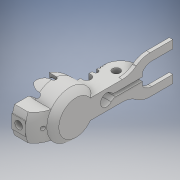
# Autodesk Inventor part: NeuroprobeholdermajigerV11MiniscopeAngle43DScope
Saved by Autodesk Inventor 2017 (Build 210142000, 142)
## iProperties
Created: 2017-09-22
Part Number: NeuroprobeholdermajigerV11MiniscopeAngle43DScope
Material: Generic
Document SubType Name: Modeling
Designer: andrew
Density: 1 g/cm^3
Appearance: Default
Author: andrew
Autodesk Inventor part; units mm, degrees
ref_plane "YZ Plane" through (0, 0, 0) normal (1, 0, 0) x (0, 1, 0)
sketch "Sketch2" plane through (0, 0, 0) normal (0, 0, 1) x (1, 0, 0)
  arc A0 (10.5, 0) -> (-2.9904, 10.0652) centre (0, 0) ccw
  arc A1 (0, 12) -> (-6, 10.3923) centre (0, 0) ccw
  line L0 (-5.25, 9.0933) -> (-6, 10.3923)
  line L1 (0, 0) -> (17.0475, 0) construction
  line L2 (0, 0) -> (-8.3214, 0)
  line L3 (11.5, 0) -> (0, 0)
  line L4 (0, 12) -> (8.279, 12)
  line L5 (11.5, 8.9606) -> (11.5, 0)
  line L6 (8.279, 12) -> (7.279, 12)
  line L7 (7.279, 12) -> (8.279, 12)
  arc A2 (11.5, 8.9606) -> (8.279, 12) centre (0, 0) ccw
  arc A3 (-5.25, 9.0933) -> (-4.1869, 9.0866) centre (-4.7167, 9.3682) ccw
  arc A4 (-2.9904, 10.0652) -> (-4.1869, 9.0866) centre (-2.4208, 8.148) ccw
  point P0 (-8.5237, 14.7636)
  point P1 (-8.5237, -14.7636)
  dimension "d5" = 24
  dimension "d6" = 120
  dimension "d75" = 2
  constraints: 16 end point, 10 point on circle, 5 centre point, 3 coincident, 3 horizontal, 3 point on line, 2 tangent, 1 collinear, 1 perpendicular, 1 symmetric about line
  measures "d5" diameter of A1
  measures "d6" angle of L1 L0
  measures "d75" radius of A4
revolve "Revolution2" add sketch "Sketch2" angle 360 about axis through (0, 0, 0) along (-1, 0, 0)
sketch "Sketch1" plane through (0, 0, 0) normal (0, 1, 0) x (-1, 0, 0)
  arc A0 (-10, 0) -> (9.4843, -3.17) centre (0, 0) ccw
  line L0 (0, 0) -> (0, -3.17)
  line L1 (9.4843, -3.17) -> (37.7274, -3.17)
  line L2 (0, 0) -> (4.0481, 0)
  line L3 (4.0481, 0) -> (4.0481, 0)
  line L4 (37.7274, 0) -> (37.7274, -3.17)
  line L5 (37.7274, 0) -> (-10, 0)
  point P0 (37.7274, 3.17)
  dimension "d0" = 20
  dimension "d1" = 3.17
  dimension "d2" = 90
  constraints: 12 end point, 2 perpendicular, 2 point on circle, 1 centre point, 1 coincident, 1 horizontal, 1 point on line, 1 symmetric about line, 1 vertical
  measures "d0" diameter of A0
  measures "d1" distance of L0.start L0.end
  measures "d2" angle of L1 L0
revolve "Revolution1" [suppressed]
sketch "Sketch4" plane through (0, 0, 0) normal (0, 1, 0) x (-1, 0, 0)
  line L0 (6.0157, -10.3923) -> (6.0157, 10.3923)
  line L1 (6.0157, -3.519) -> (6.0157, 3.519)
  line L2 (6, 0) -> (6, 0) construction
  line L3 (0.822, 9.7784) -> (0.822, -9.9241) construction
  arc A0 (0.0051, 1.2595) -> (6.0157, 3.519) centre (-0.0738, 10.5936) ccw
  arc A1 (-3.157, 1.9433) -> (-2.378, 1.548) centre (-1.8843, 3.4861) ccw
  arc A2 (0.0051, 1.2595) -> (0.0051, -1.2595) centre (0.0157, 0) ccw
  line L4 (-4.7599, 0) -> (0.0157, 0) construction
  arc A3 (-2.378, -1.548) -> (-3.157, -1.9433) centre (-1.8843, -3.4861) ccw
  arc A4 (6.0157, -3.519) -> (0.0051, -1.2595) centre (-0.0738, -10.5936) ccw
  line L5 (0.0157, 0) -> (-9.5355, 0) construction
  arc A5 (-3.157, 1.9433) -> (-3.157, -1.9433) centre (-4.7599, 0) ccw
  line L6 (11.1937, 0) -> (13.2584, 0)
  point P0 (0, 0)
  constraints: 12 end point, 12 point on circle, 6 centre point, 2 coincident, 1 collinear, 1 horizontal, 1 point on line, 1 vertical
extrude "Extrusion2" cut sketch "Sketch4" along normal blind 25
pattern_circular "Circular Pattern1" count 4 over 360 about axis through (-10, 0, 0) along (1, 0, 0) of "Extrusion2"
ref_plane "Work Plane1" through (0, -12, 0) normal (0, 1, 0) x (-1, 0, 0)
sketch "Sketch7" plane through (0, -12, 0) normal (0, 1, 0) x (-1, 0, 0)
  circle A0 centre (0, 0) radius 2.0066
  line L0 (-8.2285, 6.985) -> (3.5053, 6.985)
  line L1 (-8.279, -6.985) -> (3.5053, -6.985)
  line L2 (3.5053, -4.064) -> (-1.7598, -4.064)
  line L3 (-4.3994, -2.54) -> (-1.7598, -4.064)
  line L4 (-4.3994, 2.54) -> (-4.3994, -2.54)
  line L5 (-1.7598, 4.064) -> (-4.3994, 2.54)
  line L6 (-1.7598, 4.064) -> (3.5053, 4.064)
  circle A1 centre (0, 0) radius 2.0066
  line L7 (3.5053, 0.0727) -> (3.5053, 21.7197)
  line L8 (3.5053, 21.7197) -> (3.5053, -17.1959)
  line L9 (-8.279, -6.985) -> (-8.279, 6.985)
  line L10 (-8.2285, 6.985) -> (-8.279, 6.985)
  point P0 (0, 0)
  point P1 (0, 0)
  constraints: 22 end point, 5 point on line, 2 centre point
extrude "Extrusion4" add sketch "Sketch7" along normal blind 1.5
sketch "Sketch8" plane through (0, -10.5, 0) normal (0, 1, 0) x (1, 0, 0)
  line L0 (0, -5.8095) -> (8.279, -5.8095) projected
  arc A0 (-3.5053, -4.6328) -> (0, -5.8095) centre (0, 0) ccw projected
  line L1 (-3.5053, -4.6328) -> (-3.5053, -6.985) projected
  line L2 (-3.5053, -6.985) -> (8.279, -6.985) projected
  line L3 (8.279, 5.8095) -> (0, 5.8095) projected
  line L4 (8.279, 6.985) -> (-3.5053, 6.985) projected
  line L5 (-3.5053, 6.985) -> (-3.5053, 4.6328) projected
  arc A1 (0, 5.8095) -> (-3.5053, 4.6328) centre (0, 0) ccw projected
  line L6 (8.279, 5.8095) -> (8.279, 6.985) projected
  line L7 (8.279, -6.985) -> (8.279, -5.8095) projected
extrude "Extrusion5" add sketch "Sketch8" along normal blind 1.5
sketch "Sketch9" plane through (0, -12, 0) normal (0, -1, 0) x (1, 0, 0)
  circle A0 centre (0, 0) radius 2.0066
  line L0 (-3.5053, 6.985) -> (3.5053, 6.985)
  line L1 (-3.5053, -6.985) -> (3.5053, -6.985)
  line L2 (1.7598, -4.064) -> (-1.7598, -4.064)
  line L3 (-1.7598, 4.064) -> (1.7598, 4.064)
  circle A1 centre (0, 0) radius 2.0066
  circle A2 centre (0, 0) radius 2.0066
  line L4 (5.4916, 6.985) -> (-3.5053, 6.985)
  line L5 (5.4916, -6.985) -> (-3.5053, -6.985)
  line L6 (-3.5053, -4.064) -> (1.7598, -4.064)
  line L7 (4.3994, -2.54) -> (1.7598, -4.064)
  line L8 (4.3994, 2.54) -> (4.3994, -2.54)
  line L9 (1.7598, 4.064) -> (4.3994, 2.54)
  line L10 (1.7598, 4.064) -> (-3.5053, 4.064)
  circle A3 centre (0, 0) radius 2.0066
  line L11 (-3.5053, 0.0727) -> (-3.5053, 6.985)
  line L12 (-3.5053, 6.985) -> (-3.5053, -6.985)
  line L13 (8.279, 6.985) -> (5.6673, 6.985)
  line L14 (-3.5053, 6.985) -> (8.279, 6.985) projected
  line L15 (8.279, -6.985) -> (-3.5053, -6.985) projected
  line L16 (5.4916, -6.985) -> (8.279, -6.985)
  line L17 (8.279, 6.985) -> (8.279, -6.985)
  point P0 (0, 0)
  point P1 (0, 0)
  point P2 (-3.5053, -17.1959)
  constraints: 32 end point, 5 point on line, 4 centre point, 1 horizontal, 1 vertical
extrude "Extrusion6" add sketch "Sketch9" along normal blind 3.302 contours L0 L4 L14 L13 L17 L15 L5 L1 L12 L6 L2 L7 L8 L9 L3 L10 L11
sketch "Sketch10" plane through (0, -15.302, 0) normal (0, -1, 0) x (1, 0, 0)
  circle A0 centre (0, 0) radius 2.0066
  line L0 (-3.5053, 6.985) -> (3.5053, 6.985)
  line L1 (-3.5053, -6.985) -> (3.5053, -6.985)
  line L2 (1.7598, -4.064) -> (-1.7598, -4.064)
  line L3 (-1.7598, 4.064) -> (1.7598, 4.064)
  circle A1 centre (0, 0) radius 2.0066
  line L4 (-3.5053, 0.0727) -> (-3.5053, 6.985)
  line L5 (1.7598, 4.064) -> (-3.5053, 4.064)
  line L6 (1.7598, 4.064) -> (4.3994, 2.54)
  line L7 (5.4916, 6.985) -> (-3.5053, 6.985)
  line L8 (-3.5053, 6.985) -> (-3.5053, -6.985)
  circle A2 centre (0, 0) radius 2.0066
  line L9 (4.3994, 2.54) -> (4.3994, -2.54)
  line L10 (-3.5053, -4.064) -> (1.7598, -4.064)
  line L11 (4.3994, -2.54) -> (1.7598, -4.064)
  line L12 (5.4916, -6.985) -> (-3.5053, -6.985)
  circle A3 centre (0, 0) radius 2.0066
  line L13 (8.279, -6.985) -> (0, -6.985) projected
  line L14 (5.4916, -6.985) -> (8.279, -6.985)
  line L15 (8.279, -6.985) -> (8.279, 6.985)
  line L16 (8.279, 6.985) -> (5.4916, 6.985)
  line L17 (0, 6.985) -> (8.279, 6.985) projected
  point P0 (0, 0)
  point P1 (0, 0)
  point P2 (-3.5053, -17.1959)
  constraints: 32 end point, 4 centre point, 4 point on line, 2 collinear, 1 perpendicular
extrude "Extrusion7" add sketch "Sketch10" along normal blind 3.048
ref_plane "Work Plane3" through (0, 0, 0) normal (0, -0.7071068, 0.7071068) x (1, 0, 0)
sketch "Sketch12" plane through (0, 0, 0) normal (0, -0.7071068, 0.7071068) x (1, 0, 0)
  line L0 (-6.0157, 3.519) -> (-6.0157, -3.519)
  line L1 (-6.0157, 10.3923) -> (-6.0157, -10.3923)
  line L2 (-6, 0) -> (-6, 0) construction
  line L3 (-0.822, -9.7784) -> (-0.822, 9.9241) construction
  arc A0 (3.157, -1.9433) -> (2.378, -1.548) centre (1.8843, -3.4861) ccw
  arc A1 (2.378, 1.548) -> (3.157, 1.9433) centre (1.8843, 3.4861) ccw
  arc A2 (3.157, -1.9433) -> (3.157, 1.9433) centre (4.7599, 0) ccw
  line L4 (-0.0157, 0) -> (9.5355, 0) construction
  line L5 (4.7599, 0) -> (-0.0157, 0) construction
  arc A3 (0, -1.2594) -> (-6.0157, -3.519) centre (0.0738, -10.5936) ccw
  arc A4 (-6.0157, 3.519) -> (0, 1.2594) centre (0.0738, 10.5936) ccw
  line L6 (-10.5976, -5.502) -> (-8.5328, -5.502)
  line L7 (-6, -4.439) -> (-6, 4.439) projected
  line L8 (-6, 4.439) -> (-6, -4.439)
  line L9 (-6, -4.439) -> (-6, 0)
  line L10 (-6, 0) -> (-10.5976, 0)
  arc A5 (-0.0102, -1.2595) -> (-0.0102, 1.2595) centre (-0.0157, 0) ccw
  point P0 (0, 0)
  point P1 (0, 0)
  constraints: 20 end point, 16 point on circle, 6 centre point, 2 coincident, 2 horizontal, 1 collinear, 1 midpoint, 1 point on line, 1 vertical
extrude "Extrusion8" cut sketch "Sketch12" against normal blind 20
pattern_circular "Circular Pattern2" count 4 over 360 about axis through (-10, 0, 0) along (1, 0, 0) of "Extrusion8"
sketch "Sketch13" plane through (0, 0, 0) normal (0, 0, 1) x (1, 0, 0)
  line L0 (8.279, -9.7575) -> (8.279, -9.7575) construction
  line L1 (8.279, -9.7575) -> (8.279, -9.7575) construction
  line L2 (11.5, -8.9606) -> (11.5, 8.9606) construction
  arc A0 (8.279, -12) -> (8.279, 12) centre (0, 0) ccw construction
  line L3 (2.0066, -15.302) -> (2.0066, -18.35) construction
  line L4 (2.0066, -18.35) -> (3.5066, -18.35) construction
  line L5 (-3.5053, -18.35) -> (8.279, -18.35) construction
  line L6 (3.5066, -18.35) -> (8.279, -12) construction
  arc A1 (3.5066, -18.35) -> (8.279, -12) centre (-1.8822, -9.3316) ccw
  line L7 (8.279, -12) -> (10.647, -12)
  line L8 (10.647, -12) -> (10.647, -21.3275)
  line L9 (10.647, -21.3275) -> (3.5066, -21.3275)
  line L10 (3.5066, -21.3275) -> (3.5066, -18.35)
  line L11 (-7.1221, 0) -> (18.1956, 0) projected
  dimension "d53" = 1.5
  constraints: 12 end point, 3 perpendicular, 2 point on circle, 1 centre point, 1 horizontal, 1 point on line
  measures "d53" distance of L3.end L4.end
revolve "Revolution3" cut sketch "Sketch13" angle 360 about axis through (-10, 0, 0) along (1, 0, 0)
sketch "Sketch14" plane through (3.5066, -18.35, -6.985) normal (1, 0, 0) x (0, 0, -1)
  line L0 (0, 1.3814) -> (0, 0) projected
  arc A0 (-6.985, 0) -> (0, 1.3814) centre (-6.985, 18.35) ccw projected
  line L1 (0, 0) -> (-6.985, 0) projected
  line L2 (-13.97, 0) -> (-13.97, 1.3814) projected
  line L3 (-6.985, 0) -> (-13.97, 0) projected
  arc A1 (-13.97, 1.3814) -> (-6.985, 0) centre (-6.985, 18.35) ccw projected
  line L4 (0, 0) -> (-6.985, 0) projected
  line L5 (-3.485, 0) -> (-3.485, 0.3369)
  line L6 (-13.97, 0) -> (0, 0) projected
  line L7 (-10.485, 0) -> (-10.485, 0.3369)
  line L8 (0, 1.3814) -> (0, 0) projected
  line L9 (0, 1.3814) -> (0, 0)
  line L10 (0, 0) -> (-3.485, 0)
  line L11 (-10.485, 0) -> (-13.97, 0)
  line L12 (-13.97, 1.3814) -> (-13.97, 0)
  arc A2 (-13.97, 1.3814) -> (-10.485, 0.3369) centre (-6.985, 18.35) ccw
  arc A3 (-3.485, 0.3369) -> (0, 1.3814) centre (-6.985, 18.35) ccw
  constraints: 12 end point, 4 point on circle, 2 centre point, 2 collinear, 2 point on line, 2 vertical, 1 perpendicular, 1 tangent
extrude "Extrusion9" cut sketch "Sketch14" against normal blind 20 contours L0 L1 L5 A0 | L3 L2 A1 L7
sketch "Sketch16" plane through (11.5, 0, 0) normal (1, 0, 0) x (0, 0, -1)
  line L0 (1.016, 20.666) -> (1.016, 29.9736)
  arc A0 (1.016, 20.666) -> (2.0941, 18.282) centre (4.191, 20.666) ccw
  arc A1 (-2.0969, 18.2844) -> (2.0941, 18.282) centre (-0.0028, 15.8979) ccw
  arc A2 (-2.0969, 18.2844) -> (-1.016, 20.6709) centre (-4.191, 20.6709) ccw
  line L1 (5.08, 24.068) -> (5.08, 7.3814)
  line L2 (7.9375, 50.4096) -> (5.75, 50.4096)
  circle A3 centre (0, 0) radius 8.9606 projected
  line L3 (5.75, 39.399) -> (5.75, 50.4096)
  line L4 (7.9375, 50.4096) -> (9.9375, 50.4096)
  line L5 (9.9375, 50.4096) -> (9.9375, 38.5471)
  line L6 (7.5923, 31.4208) -> (7.4252, 31.1944)
  arc A4 (7.5923, 31.4208) -> (9.9375, 38.5471) centre (-2.0625, 38.5471) ccw
  arc A5 (7.4252, 31.1944) -> (5.08, 24.068) centre (17.08, 24.068) ccw
  arc A6 (3.4334, 34.7865) -> (5.75, 39.399) centre (0, 39.399) ccw
  arc A7 (3.4334, 34.7865) -> (1.016, 29.9736) centre (7.016, 29.9736) ccw
  line L7 (0, 23.8596) -> (0, 28.4942)
  line L8 (-1.016, 20.6709) -> (-1.016, 29.9736)
  line L9 (-5.08, 24.068) -> (-5.08, 7.3814)
  line L10 (-7.9375, 50.4096) -> (-5.75, 50.4096)
  line L11 (-5.75, 39.399) -> (-5.75, 50.4096)
  line L12 (-7.9375, 50.4096) -> (-9.9375, 50.4096)
  line L13 (-9.9375, 50.4096) -> (-9.9375, 38.5471)
  line L14 (-7.5923, 31.4208) -> (-7.4252, 31.1944)
  arc A8 (-9.9375, 38.5471) -> (-7.5923, 31.4208) centre (2.0625, 38.5471) ccw
  arc A9 (-5.08, 24.068) -> (-7.4252, 31.1944) centre (-17.08, 24.068) ccw
  arc A10 (-5.75, 39.399) -> (-3.4334, 34.7865) centre (0, 39.399) ccw
  arc A11 (-1.016, 29.9736) -> (-3.4334, 34.7865) centre (-7.016, 29.9736) ccw
  circle A12 centre (0, 0) radius 8.9606
  point P0 (5.08, 33.717)
  point P1 (1.016, 33.7394)
  point P2 (5.08, 30.4254)
  point P3 (-1.016, 33.7394)
  point P4 (-5.08, 30.4254)
  point P5 (-5.08, 33.717)
  dimension "d86" = 2
  dimension "d87" = 12
  constraints: 30 end point, 26 point on circle, 16 symmetric about line, 11 centre point, 6 tangent, 4 point on line, 2 perpendicular, 1 coincident, 1 equal radius, 1 horizontal, 1 vertical, 7 other
  measures "d86" distance of L2.start L4.end
  measures "d87" radius of A4
extrude "Extrusion10" add sketch "Sketch16" against normal blind 1.8288 contours L0 A7 A6 L3 L2 L4 L5 A4 L6 A5 L1 A3 L9 A9 L14 A8 L13 L12 L10 L11 A10 A11 L8 A2 A1 A0
sketch "Sketch18" plane through (11.5, 7.3814, -5.08) normal (0, 0, -1) x (-1, 0, 0)
  line L0 (9.5611, 16.7122) -> (5.4916, 14.3627)
  line L1 (5.4916, 14.3627) -> (1.4222, 16.7122)
  line L2 (1.4222, 16.7122) -> (1.4222, 21.4112)
  line L3 (1.4222, 21.4112) -> (5.4916, 23.7607)
  line L4 (5.4916, 23.7607) -> (9.5611, 21.4112)
  line L5 (9.5611, 21.4112) -> (9.5611, 16.7122)
  arc A0 (11.391, 17.924) -> (11.391, 17.3707) centre (11.2352, 17.6473) ccw
  line L6 (11.391, 17.924) -> (11.391, 18.6049)
  arc A1 (11.388, 19.0728) -> (11.391, 18.6049) centre (11.2906, 18.8382) ccw
  arc A2 (11.388, 19.0728) -> (4.0749, 27.2166) centre (2.7105, 18.636) ccw
  line L7 (0, 27.2166) -> (0, 3.3936)
  line L8 (11.391, 3.3936) -> (11.391, 6.4986)
  arc A3 (11.391, 10.6375) -> (11.391, 6.4986) centre (10.4199, 8.568) ccw
  line L9 (11.391, 10.6375) -> (11.391, 12.508)
  arc A4 (11.391, 14.6698) -> (11.391, 12.508) centre (10.7243, 13.5889) ccw
  line L10 (11.391, 14.6698) -> (11.391, 15.7745)
  arc A5 (11.391, 16.5568) -> (11.391, 15.7745) centre (11.1798, 16.1657) ccw
  line L11 (11.391, 16.5568) -> (11.391, 17.3707)
  circle A6 centre (5.6186, 19.0072) radius 2.0066
  line L12 (5.4916, 23.7607) -> (9.5611, 21.4112)
  line L13 (1.4222, 21.4112) -> (5.4916, 23.7607)
  line L14 (1.4222, 16.7122) -> (1.4222, 21.4112)
  line L15 (5.4916, 14.3627) -> (1.4222, 16.7122)
  line L16 (9.5611, 16.7122) -> (5.4916, 14.3627)
  line L17 (9.5611, 21.4112) -> (9.5611, 16.7122)
  line L18 (0, 27.2166) -> (1.8444, 27.2166)
  line L19 (1.8444, 27.2166) -> (4.0749, 27.2166)
  line L20 (1.8288, 16.6866) -> (1.8288, 2.2728) projected
  line L21 (11.391, 3.3936) -> (11.391, 3.0426)
  line L22 (11.391, 3.0426) -> (0, 3.0426)
  line L23 (0, 3.0426) -> (0, 3.3936)
  point P0 (11.5, -7.3814)
  point P1 (-2.7178, 26.3356)
  point P2 (1.8288, 23.044)
  dimension "d68" = 0.4066
  dimension "d79" = 0.351
  constraints: 46 end point, 12 point on circle, 7 centre point, 2 perpendicular, 1 horizontal, 1 vertical
  measures "d68" distance between parallel lines of L20 L2
  measures "d79" distance of L8.start L21.end
extrude "Extrusion11" add sketch "Sketch18" against normal blind 10.16 contours A0 L11 A5 L10 A4 L9 A3 L8 L21 L22 L23 L7 L18 L19 A2 A1 L6
sketch "Sketch20" plane through (11.5, 7.3814, 5.08) normal (0, 0, 1) x (1, 0, 0)
  line L0 (-5.4916, 23.7607) -> (-9.5611, 21.4112) construction
  line L1 (-5.4916, 14.3627) -> (-1.8288, 16.4774) construction
  line L2 (-5.4916, 23.7607) -> (-5.4916, 14.3627) construction
  line L3 (-5.4916, 14.3627) -> (-9.5611, 16.7122)
  line L4 (-9.5611, 16.7122) -> (-9.5611, 21.4112)
  line L5 (-9.5611, 21.4112) -> (-5.4916, 23.7607)
  line L6 (-5.4916, 23.7607) -> (-1.4222, 21.4112)
  line L7 (-1.4222, 21.4112) -> (-1.4222, 16.7122)
  line L8 (-1.4222, 16.7122) -> (-5.4916, 14.3627)
  point P0 (-11.5, -7.3814)
  point P1 (-5.4916, 19.0617)
  constraints: 18 end point, 1 vertical, 13 other
extrude "Extrusion13" cut sketch "Sketch20" against normal blind 20
sketch "Sketch21" plane through (11.5, 7.3814, 5.08) normal (0, 0, 1) x (1, 0, 0)
  line L0 (9.5611, 16.7122) -> (5.4916, 14.3627)
  line L1 (5.4916, 14.3627) -> (1.4222, 16.7122)
  line L2 (9.5611, 16.7122) -> (5.4916, 14.3627)
  line L3 (5.4916, 14.3627) -> (1.4222, 16.7122)
  line L4 (9.5611, 21.4112) -> (9.5611, 16.7122)
  line L5 (1.4222, 16.7122) -> (1.4222, 21.4112)
  line L6 (1.4222, 21.4112) -> (5.4916, 23.7607)
  line L7 (5.4916, 23.7607) -> (9.5611, 21.4112)
  circle A0 centre (-5.4916, 19.0617) radius 2.0066
  line L8 (1.4222, 16.7122) -> (1.4222, 21.4112)
  line L9 (9.5611, 21.4112) -> (9.5611, 16.7122)
  line L10 (1.4222, 21.4112) -> (5.4916, 23.7607)
  line L11 (5.4916, 23.7607) -> (9.5611, 21.4112)
  line L12 (-5.4916, 14.3627) -> (-9.5611, 16.7122)
  line L13 (-5.4916, 23.7607) -> (-1.4222, 21.4112)
  line L14 (-5.4916, 14.3627) -> (-5.4916, 23.7607) construction
  line L15 (-5.4916, 19.0617) -> (-7.5263, 19.0617) construction
  line L16 (-9.5611, 16.7122) -> (-9.5611, 21.4112)
  line L17 (-9.5611, 21.4112) -> (-5.4916, 23.7607)
  line L18 (-1.4222, 21.4112) -> (-1.4222, 16.7122)
  line L19 (-1.4222, 16.7122) -> (-5.4916, 14.3627)
  point P0 (-11.5, -7.3814)
  point P1 (11.5, -7.3814)
  constraints: 40 end point, 1 centre point, 1 horizontal, 1 midpoint, 1 vertical
extrude "Extrusion14" add sketch "Sketch21" against normal blind 8.382 contours L12 L16 L17 L13 L18 L19
sketch "Sketch19" plane through (11.5, 38.5471, 9.9375) normal (1, 0, 0) x (0, 0, -1)
  line L0 (8.9215, -3.9491) -> (8.9215, -17.8762)
  line L1 (10.9535, -17.8811) -> (10.9535, -3.9491)
  arc A0 (7.8406, -20.2627) -> (8.9215, -17.8762) centre (5.7465, -17.8762) ccw
  arc A1 (10.9535, -17.8811) -> (12.0316, -20.2651) centre (14.1285, -17.8811) ccw
  line L2 (4.8575, -31.1657) -> (4.8575, -8.1217)
  line L3 (15.0175, -8.1217) -> (15.0175, -31.1657)
  arc A2 (7.8406, -20.2627) -> (12.0316, -20.2651) centre (9.9347, -22.6492) ccw
  arc A3 (4.8575, -8.1217) -> (3.9276, -5.8766) centre (1.6825, -8.1217) ccw
  line L4 (3.9276, -5.8766) -> (2, -3.9491)
  line L5 (15.9474, -5.8766) -> (17.875, -3.9491)
  arc A4 (10.9535, -3.9491) -> (14.065, -0.7747) centre (10.89, -0.7747) ccw
  arc A5 (5.81, -0.7747) -> (8.9215, -3.9491) centre (8.985, -0.7747) ccw
  line L6 (2, -3.9491) -> (2, 11.8624)
  line L7 (2, 11.8624) -> (5.81, 11.8624)
  line L8 (5.81, 11.8624) -> (5.81, -0.7747)
  line L9 (14.065, 11.8624) -> (14.065, -0.7747)
  line L10 (17.875, -3.9491) -> (17.875, 11.8624)
  line L11 (17.875, 11.8624) -> (14.065, 11.8624)
  arc A6 (15.9474, -5.8766) -> (15.0175, -8.1217) centre (18.1925, -8.1217) ccw
  circle A7 centre (9.9375, -38.5471) radius 8.9606
  line L12 (5.81, 11.8624) -> (2, 11.8624)
  line L13 (14.065, 11.8624) -> (5.81, 11.8624)
  arc A8 (6.7443, -3.9491) -> (6.5041, -3.7606) centre (2.9215, -8.5736) ccw construction
  arc A9 (4.1875, 0.8519) -> (6.5041, -3.7606) centre (9.9375, 0.8519) ccw construction
  line L14 (4.1875, 0.8519) -> (4.1875, 11.8624) construction
  line L15 (4.1875, 11.8624) -> (0, 11.8624) construction
  line L16 (0, 11.8624) -> (0, 0) construction
  arc A10 (0, 0) -> (2.3452, -7.1263) centre (12, 0) ccw construction
  line L17 (2.3452, -7.1263) -> (2.5123, -7.3528) construction
  arc A11 (4.8575, -14.4791) -> (2.5123, -7.3528) centre (-7.1425, -14.4791) ccw construction
  line L18 (4.8575, -14.4791) -> (4.8575, -31.1657) construction
  arc A12 (4.8575, -31.1657) -> (15.0175, -31.1657) centre (9.9375, -38.5471) ccw construction
  line L19 (15.0175, -31.1657) -> (15.0175, -14.4791) construction
  arc A13 (17.3627, -7.3528) -> (15.0175, -14.4791) centre (27.0175, -14.4791) ccw construction
  line L20 (17.3627, -7.3528) -> (17.5298, -7.1263) construction
  arc A14 (17.5298, -7.1263) -> (19.875, 0) centre (7.875, 0) ccw construction
  line L21 (19.875, 0) -> (19.875, 11.8624) construction
  line L22 (19.875, 11.8624) -> (15.6875, 11.8624) construction
  line L23 (15.6875, 11.8624) -> (15.6875, 0.8519) construction
  arc A15 (13.3709, -3.7606) -> (15.6875, 0.8519) centre (9.9375, 0.8519) ccw construction
  arc A16 (13.3709, -3.7606) -> (13.1307, -3.9491) centre (16.9535, -8.5736) ccw construction
  line L24 (13.1307, -3.9491) -> (6.7443, -3.9491) construction
  point P0 (9.9375, -38.5471)
  point P1 (9.9375, -38.5471)
  point P2 (15.0175, -4.8301)
  constraints: 28 end point, 16 point on circle, 8 centre point, 1 horizontal
extrude "Extrusion12" cut sketch "Sketch19" against normal blind 20 contours A5 L8 L13 L9 A4 L1 A1 A2 A0 L0
sketch "Sketch22" plane through (4.3994, -12, -2.54) normal (-1, 0, 0) x (0, 0, 1)
  circle A0 centre (2.54, -1.5109) radius 1
  point P0 (2.54, 12)
  dimension "d76" = 2
  constraints: 1 centre point
  measures "d76" diameter of A0
extrude "Extrusion15" cut sketch "Sketch22" against normal blind 10
sketch "Sketch23" plane through (8.836, 10.424, -5.08) normal (0, -1, 0) x (1, 0, 0)
  line L0 (0.8352, 1.8629) -> (0.8352, 0) projected
  arc A0 (0, 0) -> (0.8352, 1.8629) centre (-8.836, 5.08) ccw projected
  line L1 (0.8352, 0) -> (0, 0) projected
  arc A1 (0.8352, 8.2971) -> (0, 10.16) centre (-8.836, 5.08) ccw projected
  line L2 (0.8352, 1.8629) -> (0.8352, 0) projected
  line L3 (0, 10.16) -> (0.8352, 10.16) projected
  arc A2 (0, 0) -> (0.8352, 1.8629) centre (-8.836, 5.08) ccw projected
  line L4 (0.8352, 0) -> (0, 0) projected
  line L5 (0.8352, 10.16) -> (0.8352, 8.2971) projected
extrude "Extrusion16" add sketch "Sketch23" along normal blind 2
body "Solid1"
